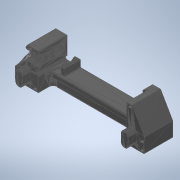
# Autodesk Inventor part: Vise_Base_A
Saved by Autodesk Inventor 2021.2 (Build 252289000, 289)
## iProperties
Created: 2021-03-05
Part Number: Vise_Base_A
Material: Generic
Document SubType Name: Modeling
Designer: robst
Density: 1 g/cm^3
Appearance: Default
Author: robst
Autodesk Inventor part; units mm, degrees
ref_plane "YZ Plane" through (0, 0, 0) normal (1, 0, 0) x (0, 1, 0)
ref_plane "XZ Plane" through (0, 0, 0) normal (0, 1, 0) x (-1, 0, 0)
ref_plane "XY Plane" through (0, 0, 0) normal (0, 0, 1) x (1, 0, 0)
sketch "Sketch2" plane through (5, -18, -18.325) normal (0, -1, 0.0000001) x (1, 0, 0)
  line L0 (-33.4327, -16.375) -> (123.4327, -16.375) projected
  line L1 (0, 0.8) -> (96.975, 0.8) projected
  line L2 (123.0111, 18.325) -> (123.0111, -16.675) projected
  line L3 (-33.0111, -16.675) -> (-33.0111, 18.325) projected
  line L4 (96.975, 0.8) -> (0, 0.8)
  line L5 (0, 0.8) -> (0, -16.375)
  line L6 (0, -16.375) -> (96.975, -16.375)
  line L7 (96.975, -16.375) -> (96.975, 0.8)
  point P0 (-5, 18.325)
  point P1 (0, 0.8)
  constraints: 8 end point, 2 parallel, 1 horizontal, 1 perpendicular, 1 point on line
extrude "Extrusion1" add sketch "Sketch2" against normal blind 0.425
sketch "Sketch3" plane through (5, -18, -18.325) normal (0, -1, 0.0000001) x (1, 0, 0)
  line L0 (0, -16.375) -> (96.975, -16.375) projected
  line L1 (0, 0.8) -> (0, -16.375) projected
  line L2 (96.975, 0.8) -> (0, 0.8) projected
  line L3 (96.975, -16.375) -> (96.975, 0.8) projected
  line L4 (0, -16.375) -> (0, 0.8) construction
  line L5 (0, -7.7875) -> (96.975, -7.7875) construction
  line L6 (96.975, 0.8) -> (96.975, -16.375) construction
  point P0 (-5, 18.325)
  point P1 (10, -7.7875)
  point P2 (86.975, -7.7875)
  dimension "d2" = 10
  dimension "d3" = 10
  constraints: 2 end point, 2 midpoint, 2 point on line
  measures "d2" distance from line of point (10, -7.787) L1
  measures "d3" distance of point (86.975, -7.787) L5.end
hole "Hole1" at (15, -18, -26.1125) at (91.975, -18, -26.1125) direction (0, 1, -0.0000001) diameter 7.9248 end through all counterbore diameter 8.0264 counterbore depth 7.4168
body "Solid1"
